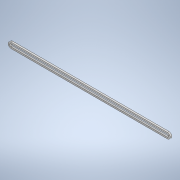
# Autodesk Inventor part: 零件4
Saved by Autodesk Inventor 2022.3 (Build 263350000, 350)
## iProperties
Created: 2023-04-16
Part Number: 零件4
Material: 一般
Document SubType Name: Modeling
Designer: JOU
Density: 1 g/cm^3
Appearance: 預設
Author: JOU
Autodesk Inventor part; units mm, degrees
ref_plane "YZ Plane" through (0, 0, 0) normal (1, 0, 0) x (0, 1, 0)
ref_plane "XZ Plane" through (0, 0, 0) normal (0, 1, 0) x (-1, 0, 0)
ref_plane "XY Plane" through (0, 0, 0) normal (0, 0, 1) x (1, 0, 0)
sketch "草圖1" plane through (0, 0, 0) normal (0, 0, 1) x (1, 0, 0)
  line L0 (-140, 0) -> (140, 0) construction
  line L1 (-140, 2.3) -> (140, 2.3)
  line L2 (140, -2.3) -> (-140, -2.3)
  arc A0 (-140, 2.3) -> (-140, -2.3) centre (-140, 0) ccw
  arc A1 (140, -2.3) -> (140, 2.3) centre (140, 0) ccw
  line L3 (-140, 0) -> (140, 0) construction
  line L4 (-140, -5) -> (140, -5)
  line L5 (140, 5) -> (-140, 5)
  arc A2 (-140, 5) -> (-140, -5) centre (-140, 0) ccw
  arc A3 (140, -5) -> (140, 5) centre (140, 0) ccw
  point P0 (0, 0)
  point P1 (0, 0)
  point P2 (0, 0)
  dimension "d5" = 5
  dimension "d6" = 2.3
  dimension "d7" = 280
  constraints: 16 end point, 8 point on circle, 8 tangent, 4 centre point, 2 coincident, 2 midpoint, 2 parallel, 2 point on line, 2 vertical alignment, 1 horizontal
  measures "d5" radius of A2
  measures "d6" radius of A0
  measures "d7" distance of L3.end L3.start
extrude "擠出1" add sketch "草圖1" along normal blind 3
